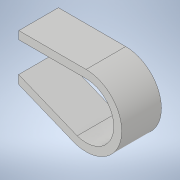
# Autodesk Inventor part: 01_Laser_Clamp_OnOffSwitch
Saved by Autodesk Inventor 2022 (Build 260153000, 153)
## iProperties
Created: 2019-05-07
Part Number: 01_Laser_Clamp_OnOffSwitch
Material: Generic
Document SubType Name: Modeling
Designer: diederichbenedict
Density: 1 g/cm^3
Appearance: Default
Author: diederichbenedict
Autodesk Inventor part; units mm, degrees
ref_plane "YZ Plane" through (0, 0, 0) normal (1, 0, 0) x (0, 1, 0)
ref_plane "XZ Plane" through (0, 0, 0) normal (0, 1, 0) x (-1, 0, 0)
ref_plane "XY Plane" through (0, 0, 0) normal (0, 0, 1) x (1, 0, 0)
sketch "Sketch1" plane through (0, 0, 0) normal (0, 0, 1) x (1, 0, 0)
  circle A0 centre (0, 0) radius 6.6 projected
  line L0 (-5.743, 8.6) -> (11.2315, 8.6)
  arc A1 (8.2853, -8.9041) -> (11.2315, 8.6) centre (11.2315, -0.4) ccw
  line L1 (8.2853, -8.9041) -> (-5.7832, -3.1804)
  line L2 (-5.743, 6.6) -> (11.2315, 6.6)
  arc A2 (8.9869, -7.0304) -> (11.2315, 6.6) centre (11.2315, -0.4) ccw
  line L3 (8.9869, -7.0304) -> (-5.7832, -1.0212)
  line L4 (-5.743, 8.6) -> (-5.743, 6.6)
  line L5 (-5.7832, -1.0212) -> (-5.7832, -3.1804)
  point P0 (0, 0)
  dimension "d1" = 13.2
  dimension "d0" = 7
  dimension "d2" = 2
  dimension "d3" = 90
  constraints: 12 end point, 4 point on circle, 2 centre point, 2 horizontal, 1 parallel, 1 tangent, 4 other
  measures "d0" radius of A2
  measures "d2" distance between parallel lines of L2 L0
  measures "d3" angle of L0 L4
extrude "Extrusion1" add sketch "Sketch1" along normal blind 10 contours L2 L4 L0 A1 L1 A0 L3 A2 | A0 L1 L5 L3
body "Solid1"
